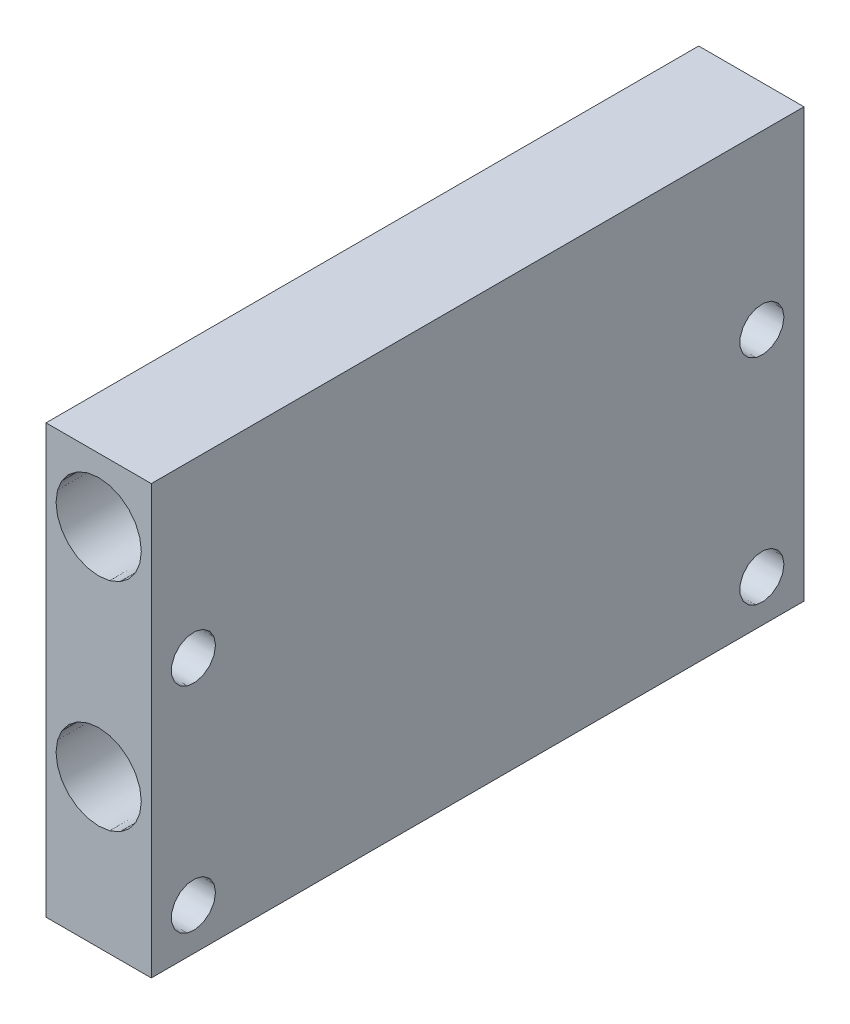
# Autodesk Inventor part: GrabberAdapterToCarbon
Saved by Autodesk Inventor 2023 (Build 270158000, 158)
## iProperties
Created: 2022-11-10
Part Number: GrabberAdapterToCarbon
Material: Generic
Document SubType Name: Modeling
Designer: deli
Density: 1 g/cm^3
Appearance: Default
Author: deli
Autodesk Inventor part; units mm, degrees
ref_plane "YZ Plane" through (0, 0, 0) normal (1, 0, 0) x (0, 1, 0)
ref_plane "XZ Plane" through (0, 0, 0) normal (0, 1, 0) x (-1, 0, 0)
ref_plane "XY Plane" through (0, 0, 0) normal (0, 0, 1) x (1, 0, 0)
sketch "Sketch1" plane through (0, 0, 0) normal (0, 0, 1) x (1, 0, 0)
  circle A0 centre (-46.4499, 27.7763) radius 4.05
  circle A1 centre (-46.4499, 7.2023) radius 4.05
  line L0 (-51.4499, 33.8263) -> (-41.4499, 33.8263)
  line L1 (-41.4499, 33.8263) -> (-41.4499, -6.8477)
  line L2 (-41.4499, -6.8477) -> (-51.4499, -6.8477)
  line L3 (-51.4499, -6.8477) -> (-51.4499, 33.8263)
  point P0 (0, 0)
  dimension "d0" = 8.1
  dimension "d1" = 20.574
  dimension "d2" = 10
  dimension "d3" = 5
  dimension "d4" = 5
  dimension "d5" = 10
  dimension "d6" = 2
  constraints: 8 end point, 2 centre point, 2 parallel, 1 equal radius, 1 horizontal, 1 perpendicular
  measures "d0" diameter of A0
  measures "d1" distance of A1.centre A0.centre
  measures "d2" distance of L1.end L2.end
  measures "d3" distance from line of A1.centre L3
  measures "d4" distance from line of L3 A0.centre
  measures "d5" distance edge to line of A1 L2
  measures "d6" distance edge to line of A0 L0
extrude "Extrusion1" add sketch "Sketch1" along normal blind 62
sketch "Sketch2" plane through (-41.4499, -6.8477, 0) normal (1, 0, 0) x (0, 0, -1)
  circle A0 centre (-58, 4) radius 2.1
  circle A1 centre (-4, 4) radius 2.1
  line L0 (-62, 0) -> (-62, 40.674) projected
  line L1 (0, 0) -> (-62, 0) projected
  line L2 (0, 0) -> (0, 40.674) projected
  circle A2 centre (-58, 24.337) radius 2.1
  circle A3 centre (-4, 24.337) radius 2.1
  line L3 (0, 40.674) -> (-62, 40.674) projected
  point P0 (0, 6.8477)
  dimension "d9" = 4.2
  dimension "d10" = 4
  dimension "d11" = 4
  dimension "d12" = 4
  dimension "d13" = 4
  dimension "d14" = 4
  dimension "d15" = 4
  dimension "d16" = 16.337
  dimension "d17" = 16.337
  constraints: 4 centre point, 3 equal radius
  measures "d9" diameter of A0
  measures "d10" distance from line of L0 A0.centre
  measures "d11" distance from line of L1 A0.centre
  measures "d12" distance from line of L1 A1.centre
  measures "d13" distance from line of L2 A1.centre
  measures "d14" distance from line of L0 A2.centre
  measures "d15" distance from line of L2 A3.centre
  measures "d16" distance from line of L3 A2.centre
  measures "d17" distance from line of L3 A3.centre
extrude "Extrusion2" cut sketch "Sketch2" against normal blind 62 contours A0 | A1 | A2 | A3
equation "\"d3\" = 0.5 * d2"
equation "\"d4\" = d3"
equation "\"d11\" = d10"
equation "\"d12\" = d10"
equation "\"d13\" = d10"
equation "\"d14\" = d10"
equation "\"d15\" = d10"
equation "\"d17\" = d16"
body "Solid1"
